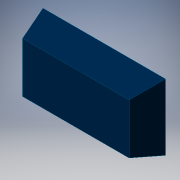
# Autodesk Inventor part: ColemanPool
Saved by Autodesk Inventor 2019 (Build 230136000, 136)
## iProperties
Created: 2021-06-08
Part Number: ColemanPool
Material: Generic
Document SubType Name: Modeling
Designer: jamieson-bl
Density: 1 g/cm^3
Appearance: Default
Author: jamieson-bl
Autodesk Inventor part; units mm, degrees
ref_plane "YZ Plane" through (0, 0, 0) normal (1, 0, 0) x (0, 1, 0)
ref_plane "XZ Plane" through (0, 0, 0) normal (0, 1, 0) x (-1, 0, 0)
sketch "Sketch1" plane through (0, 0, 0) normal (0, 0, 1) x (1, 0, 0)
  line L0 (2628.9, -1422.4) -> (-2628.9, -1422.4)
  line L1 (-2628.9, -1422.4) -> (-2628.9, 1422.4)
  line L2 (-2628.9, 1422.4) -> (2628.9, 1422.4)
  line L3 (2628.9, 1422.4) -> (2628.9, -1422.4)
  line L4 (2628.9, -1422.4) -> (-2628.9, 1422.4) construction
  line L5 (-2628.9, -1422.4) -> (2628.9, 1422.4) construction
  point P0 (0, 0)
  dimension "d0" = 5257.8
  dimension "d1" = 2844.8
  constraints: 12 end point, 2 midpoint, 2 parallel, 1 horizontal, 1 perpendicular
  measures "d0" distance of L1.end L2.end
  measures "d1" distance of L0.end L1.end
ref_plane "Work Plane1" through (0, 0, 1219.2) normal (0, 0, 1) x (1, 0, 0)
sketch "Sketch2" plane through (0, 0, 1219.2) normal (0, 0, 1) x (1, 0, 0)
  line L0 (-2286, -1079.5) -> (2286, -1079.5)
  line L1 (2286, -1079.5) -> (2286, 1079.5)
  line L2 (2286, 1079.5) -> (-2286, 1079.5)
  line L3 (-2286, 1079.5) -> (-2286, -1079.5)
  line L4 (-2286, -1079.5) -> (2286, 1079.5) construction
  line L5 (2286, -1079.5) -> (-2286, 1079.5) construction
  point P0 (0, 0)
  dimension "d3" = 4572
  dimension "d4" = 2159
  constraints: 12 end point, 2 midpoint, 2 parallel, 1 horizontal, 1 perpendicular
  measures "d3" distance of L2.end L1.end
  measures "d4" distance of L1.end L0.end
loft "Loft1" add profiles "Sketch1", "Sketch2"
body "Solid1"
